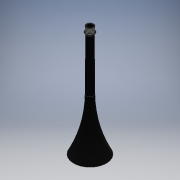
# Autodesk Inventor part: Horn_A
Saved by Autodesk Inventor 2016 (Build 200138000, 138)
## iProperties
Created: 2016-05-21
Part Number: Horn_A
Material: Steel, Cast
Document SubType Name: Modeling
Designer: agmle
Density: 7.85 g/cm^3
Appearance: Glossy - Black
Mass: 385.933 g
Surface Area: 642.869 cm^2
Volume: 49.1635 cm^3
Bell_Thickness: 1.500 mm
Flare_Length: 150.000 mm
Transition_Diameter: 10.500 mm
Flare_Diameter: 47.150 mm
Mount_Length: 15.300 mm
Mount_Diameter: 10.500 mm
Mount_Flange_Length: 5.500 mm
Mount_Flange_Diameter: 12.600 mm
Tail_Diameter: 9.500 mm
Author: agmle
Autodesk Inventor part; units mm, degrees
ref_plane "YZ Plane" through (0, 0, 0) normal (1, 0, 0) x (0, 1, 0)
ref_plane "XZ Plane" through (0, 0, 0) normal (0, 1, 0) x (-1, 0, 0)
ref_plane "XY Plane" through (0, 0, 0) normal (0, 0, 1) x (1, 0, 0)
sketch "Sketch1" plane through (0, 0, 0) normal (0, 1, 0) x (-1, 0, 0)
  line L0 (0, 0) -> (0, -320.8) construction
  line L1 (0, -320.8) -> (47.15, -320.8) construction
  line L2 (0, -170.8) -> (10.5, -170.8) construction
  line L3 (0, -20.8) -> (9.5, -20.8) construction
  line L4 (0, -15.3) -> (12.6, -15.3) construction
  line L5 (0, 0) -> (10.5, 0) construction
  line L6 (10.5, 0) -> (10.5, -15.3)
  line L7 (12.6, -15.3) -> (9.5, -20.8)
  line L8 (12.6, -15.3) -> (10.5, -15.3)
  line L9 (10.5, -170.8) -> (9.5, -20.8)
  arc A0 (10.5, -170.8) -> (47.15, -320.8) centre (344.907, -168.5706) ccw
  line L10 (7.8613, 0) -> (9, -170.8)
  arc A1 (9, -170.8) -> (45.4663, -320.8) centre (344.907, -168.5706) ccw
  line L11 (10.5, 0) -> (7.8613, 0)
  arc A2 (45.4663, -320.8) -> (47.15, -320.8) centre (46.3082, -320.372) ccw
  dimension "d0" = 47.15
  dimension "d1" = 10.5
  dimension "d2" = 9.5
  dimension "d3" = 12.6
  dimension "d4" = 10.5
  dimension "d5" = 150
  dimension "d6" = 150
  dimension "d7" = 5.5
  dimension "d8" = 15.3
  dimension "d9" = 1.5
  constraints: 24 end point, 7 point on line, 6 point on circle, 5 horizontal, 3 centre point, 2 tangent, 2 vertical, 1 collinear, 1 concentric, 1 parallel, 1 perpendicular
  measures "d0" distance of L0.end L1.end
  measures "d1" distance of L2.start L2.end
  measures "d2" distance of L3.start L3.end
  measures "d3" distance of L4.start L4.end
  measures "d4" distance of L0.start L5.end
  measures "d5" distance between parallel lines of L2 L1
  measures "d6" distance between parallel lines of L3 L2
  measures "d7" distance between parallel lines of L4 L3
  measures "d8" distance between parallel lines of L5 L4
  measures "d9" distance between parallel lines of L10 L9
revolve "Revolution1" add sketch "Sketch1" angle 360 about axis through (0, 0, 0) along (0, 0, -1)
thread "Thread1" size "M22x3" class "6g" standard "ANSI Metric M Profile" full length
equation "\"d0\" = Flare_Diameter"
equation "\"d1\" = Transition_Diameter"
equation "\"d2\" = Tail_Diameter"
equation "\"d3\" = Mount_Flange_Diameter"
equation "\"d4\" = Mount_Diameter"
equation "\"d5\" = Flare_Length"
equation "\"d6\" = Transition_Length"
equation "\"d7\" = Mount_Flange_Length"
equation "\"d8\" = Mount_Length"
equation "\"d9\" = Bell_Thickness"
equation "\"Bell_Thickness\" = 1.5"
equation "\"Flare_Length\" = 150"
equation "\"Transition_Length\" = 150"
equation "\"Transition_Diameter\" = 10.5"
equation "\"Flare_Diameter\" = 47.15"
equation "\"Mount_Length\" = 15.3"
equation "\"Mount_Diameter\" = 10.5"
equation "\"Mount_Flange_Length\" = 5.5"
equation "\"Mount_Flange_Diameter\" = 12.6"
equation "\"Tail_Diameter\" = 9.5"
body "Solid1"
